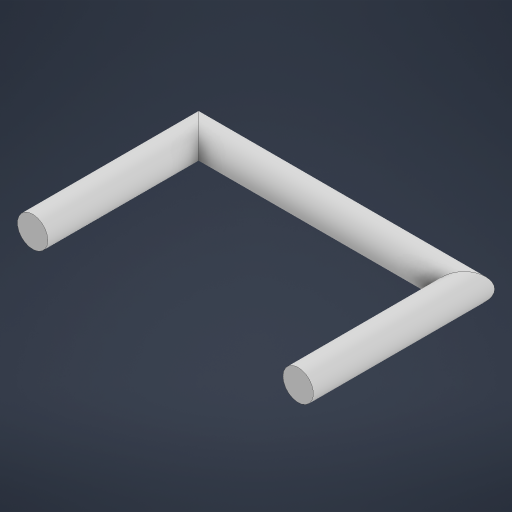
# Autodesk Inventor part: Handle
Saved by Autodesk Inventor 2024 (Build 280153000, 153)
## iProperties
Created: 2023-12-07
Part Number: Handle
Material: Generic
Document SubType Name: Modeling
Designer: calvi
Density: 1 g/cm^3
Appearance: Default
Author: calvi
Autodesk Inventor part; units mm, degrees
ref_plane "YZ Plane" through (0, 0, 0) normal (1, 0, 0) x (0, 1, 0)
ref_plane "XZ Plane" through (0, 0, 0) normal (0, 1, 0) x (-1, 0, 0)
ref_plane "XY Plane" through (0, 0, 0) normal (0, 0, 1) x (1, 0, 0)
sketch "Sketch1" plane through (0, 0, 0) normal (0, 0, 1) x (1, 0, 0)
  circle A0 centre (0, 0) radius 3.4925
  dimension "d0" = 6.985
  constraints: 1 centre point, 1 coincident
  measures "d0" diameter of A0
sketch "Sketch2" plane through (0, 0, 0) normal (0, 1, 0) x (-1, 0, 0)
  line L0 (0, 0) -> (0, -38.1)
  line L1 (0, -38.1) -> (-60.96, -38.1)
  line L2 (-60.96, -38.1) -> (-60.96, 0)
  dimension "d3" = 38.1
  dimension "d4" = 60.96
  dimension "d5" = 90
  dimension "d6" = 38.1
  dimension "d7" = 90
  constraints: 6 end point, 2 perpendicular, 1 vertical
  measures "d3" distance of L0.start L0.end
  measures "d4" distance of L0.end L1.end
  measures "d5" angle of L0 L1
  measures "d6" distance of L1.end L2.end
  measures "d7" angle of L1 L2
sweep "Sweep1" add profiles "Sketch1" path "Sketch2"
body "Solid1"
